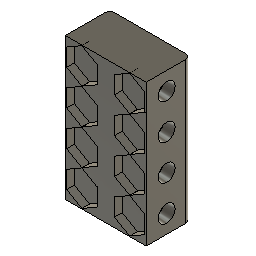
frame_rail_connector_block (Autodesk Fusion 360 archive; units mm, degrees)
design "frame connector block" references "2u(ish) rail"
Autodesk Fusion 360 part; units mm, degrees
imported_body "Derived Base Feature1" makes body 1
other "ExternalDerived1"
sketch "Sketch1" plane through (0, 0, 0) normal (0, 0, 1) x (1, 0, 0)
  arc A0 (4.25, 3.5) -> (5.75, 2) centre (5.75, 3.5) ccw
  line L0 (4.25, 3.5) -> (4.25, 14.875)
  line L1 (26, 2) -> (5.75, 2)
  arc A1 (26, 2) -> (27.5, 3.5) centre (26, 3.5) ccw
  line L2 (27.75, 3.5) -> (27.75, 14.875)
  line L3 (27.5, 14.875) -> (27.5, 3.5)
  line L4 (5.75, 14.875) -> (26, 14.875)
  line L5 (27.5, 13.375) -> (27.5, 3.5)
  line L6 (26, 2) -> (5.75, 2)
  line L7 (4.25, 3.5) -> (4.25, 13.375)
  arc A2 (4.25, 3.5) -> (5.75, 2) centre (5.75, 3.5) ccw
  arc A3 (26, 2) -> (27.5, 3.5) centre (26, 3.5) ccw
  arc A4 (5.75, 14.875) -> (4.25, 13.375) centre (5.75, 13.375) ccw
  arc A5 (27.5, 13.375) -> (26, 14.875) centre (26, 13.375) ccw
  arc A6 (27.4, 13.375) -> (26, 14.775) centre (26, 13.375) ccw
  line L8 (5.75, 14.775) -> (26, 14.775)
  arc A7 (5.75, 14.775) -> (4.35, 13.375) centre (5.75, 13.375) ccw
  line L9 (4.35, 3.5) -> (4.35, 13.375)
  arc A8 (4.35, 3.5) -> (5.75, 2.1) centre (5.75, 3.5) ccw
  line L10 (26, 2.1) -> (5.75, 2.1)
  arc A9 (26, 2.1) -> (27.4, 3.5) centre (26, 3.5) ccw
  line L11 (27.4, 13.375) -> (27.4, 3.5)
  dimension "d12" = 1.5
  dimension "d13" = 1.5
  dimension "d14" = 1.5
  dimension "d15" = 1.5
  dimension "d16" = 0.1
  constraint horizontal L4
  constraint vertical L5
  constraint horizontal L6
  constraint vertical L7
  constraint tangent L6 A2
  constraint tangent L7 A2
  constraint tangent L5 A3
  constraint tangent L6 A3
  constraint tangent L4 A4
  constraint tangent L7 A4
  constraint tangent L4 A5
  constraint tangent L5 A5
  measures "d12" radius of A2
  measures "d13" radius of A3
  measures "d14" radius of A4
  measures "d15" radius of A5
extrude "Extrude1" add sketch "Sketch1" along normal blind 40.25 separate body contours A6 L8 A7 L9 A8 L10 A9 L11 makes body 2
sketch "Sketch2" plane through (4.25, 0, 0) normal (1, 0, 0) x (0, 1, 0)
  line L0 (3.5, 0.25) -> (14.875, 0.25)
  line L1 (14.875, 0.25) -> (14.875, 130.5625)
  line L2 (14.875, 130.5625) -> (3.5, 130.5625)
  line L3 (3.5, 130.5625) -> (3.5, 0.25)
  line L4 (5.6281, 35.2188) -> (6.7828, 37.2188)
  line L5 (6.7828, 37.2188) -> (9.0922, 37.2188)
  line L6 (9.0922, 37.2188) -> (10.2469, 35.2188)
  line L7 (10.2469, 35.2188) -> (9.0922, 33.2188)
  line L8 (9.0922, 33.2188) -> (6.7828, 33.2188)
  line L9 (6.7828, 33.2188) -> (5.6281, 35.2188)
  line L10 (5.6281, 75.4688) -> (6.7828, 77.4688)
  line L11 (6.7828, 77.4688) -> (9.0922, 77.4688)
  line L12 (9.0922, 77.4688) -> (10.2469, 75.4688)
  line L13 (10.2469, 75.4688) -> (9.0922, 73.4688)
  line L14 (9.0922, 73.4688) -> (6.7828, 73.4688)
  line L15 (6.7828, 73.4688) -> (5.6281, 75.4688)
  line L16 (5.6281, 115.7188) -> (6.7828, 117.7188)
  line L17 (6.7828, 117.7188) -> (9.0922, 117.7188)
  line L18 (9.0922, 117.7188) -> (10.2469, 115.7188)
  line L19 (10.2469, 115.7188) -> (9.0922, 113.7188)
  line L20 (9.0922, 113.7188) -> (6.7828, 113.7188)
  line L21 (6.7828, 113.7188) -> (5.6281, 115.7188)
  line L22 (5.6281, 125.7813) -> (6.7828, 127.7813)
  line L23 (6.7828, 127.7813) -> (9.0922, 127.7813)
  line L24 (9.0922, 127.7813) -> (10.2469, 125.7813)
  line L25 (10.2469, 125.7813) -> (9.0922, 123.7813)
  line L26 (9.0922, 123.7813) -> (6.7828, 123.7813)
  line L27 (6.7828, 123.7813) -> (5.6281, 125.7813)
  line L28 (5.6281, 85.5313) -> (6.7828, 87.5313)
  line L29 (6.7828, 87.5313) -> (9.0922, 87.5313)
  line L30 (9.0922, 87.5313) -> (10.2469, 85.5313)
  line L31 (10.2469, 85.5313) -> (9.0922, 83.5313)
  line L32 (9.0922, 83.5313) -> (6.7828, 83.5313)
  line L33 (6.7828, 83.5313) -> (5.6281, 85.5313)
  line L34 (5.6281, 45.2813) -> (6.7828, 47.2813)
  line L35 (6.7828, 47.2813) -> (9.0922, 47.2813)
  line L36 (9.0922, 47.2813) -> (10.2469, 45.2813)
  line L37 (10.2469, 45.2813) -> (9.0922, 43.2813)
  line L38 (9.0922, 43.2813) -> (6.7828, 43.2813)
  line L39 (6.7828, 43.2813) -> (5.6281, 45.2813)
  line L40 (5.6281, 25.1563) -> (6.7828, 27.1563)
  line L41 (6.7828, 27.1563) -> (9.0922, 27.1563)
  line L42 (9.0922, 27.1563) -> (10.2469, 25.1563)
  line L43 (10.2469, 25.1563) -> (9.0922, 23.1563)
  line L44 (9.0922, 23.1563) -> (6.7828, 23.1563)
  line L45 (6.7828, 23.1563) -> (5.6281, 25.1563)
  line L46 (5.6281, 65.4063) -> (6.7828, 67.4063)
  line L47 (6.7828, 67.4063) -> (9.0922, 67.4063)
  line L48 (9.0922, 67.4063) -> (10.2469, 65.4063)
  line L49 (10.2469, 65.4063) -> (9.0922, 63.4063)
  line L50 (9.0922, 63.4063) -> (6.7828, 63.4063)
  line L51 (6.7828, 63.4063) -> (5.6281, 65.4063)
  line L52 (5.6281, 105.6563) -> (6.7828, 107.6563)
  line L53 (6.7828, 107.6563) -> (9.0922, 107.6563)
  line L54 (9.0922, 107.6563) -> (10.2469, 105.6563)
  line L55 (10.2469, 105.6563) -> (9.0922, 103.6563)
  line L56 (9.0922, 103.6563) -> (6.7828, 103.6563)
  line L57 (6.7828, 103.6563) -> (5.6281, 105.6563)
  line L58 (10.2469, 5.0313) -> (9.0922, 3.0313)
  line L59 (9.0922, 3.0313) -> (6.7828, 3.0313)
  line L60 (6.7828, 3.0313) -> (5.6281, 5.0313)
  line L61 (5.6281, 5.0313) -> (6.7828, 7.0313)
  line L62 (6.7828, 7.0313) -> (9.0922, 7.0313)
  line L63 (9.0922, 7.0313) -> (10.2469, 5.0313)
  line L64 (5.6281, 95.5938) -> (6.7828, 97.5938)
  line L65 (6.7828, 97.5938) -> (9.0922, 97.5938)
  line L66 (9.0922, 97.5938) -> (10.2469, 95.5938)
  line L67 (10.2469, 95.5938) -> (9.0922, 93.5938)
  line L68 (9.0922, 93.5938) -> (6.7828, 93.5938)
  line L69 (6.7828, 93.5938) -> (5.6281, 95.5938)
  line L70 (5.6281, 55.3438) -> (6.7828, 57.3438)
  line L71 (6.7828, 57.3438) -> (9.0922, 57.3438)
  line L72 (9.0922, 57.3438) -> (10.2469, 55.3438)
  line L73 (10.2469, 55.3438) -> (9.0922, 53.3438)
  line L74 (9.0922, 53.3438) -> (6.7828, 53.3438)
  line L75 (6.7828, 53.3438) -> (5.6281, 55.3438)
  line L76 (5.6281, 15.0938) -> (6.7828, 17.0938)
  line L77 (6.7828, 17.0938) -> (9.0922, 17.0938)
  line L78 (9.0922, 17.0938) -> (10.2469, 15.0938)
  line L79 (10.2469, 15.0938) -> (9.0922, 13.0938)
  line L80 (9.0922, 13.0938) -> (6.7828, 13.0938)
  line L81 (6.7828, 13.0938) -> (5.6281, 15.0938)
  line L82 (6.7828, 17.0938) -> (5.6281, 15.0938)
  line L83 (5.6281, 15.0938) -> (6.7828, 13.0938)
  line L84 (6.7828, 13.0938) -> (9.0922, 13.0938)
  line L85 (9.0922, 13.0938) -> (10.2469, 15.0938)
  line L86 (10.2469, 15.0938) -> (9.0922, 17.0938)
  line L87 (9.0922, 17.0938) -> (6.7828, 17.0938)
  line L88 (6.7828, 57.3438) -> (5.6281, 55.3438)
  line L89 (5.6281, 55.3438) -> (6.7828, 53.3438)
  line L90 (6.7828, 53.3438) -> (9.0922, 53.3438)
  line L91 (9.0922, 53.3438) -> (10.2469, 55.3438)
  line L92 (10.2469, 55.3438) -> (9.0922, 57.3438)
  line L93 (9.0922, 57.3438) -> (6.7828, 57.3438)
  line L94 (6.7828, 97.5938) -> (5.6281, 95.5938)
  line L95 (5.6281, 95.5938) -> (6.7828, 93.5938)
  line L96 (6.7828, 93.5938) -> (9.0922, 93.5938)
  line L97 (9.0922, 93.5938) -> (10.2469, 95.5938)
  line L98 (10.2469, 95.5938) -> (9.0922, 97.5938)
  line L99 (9.0922, 97.5938) -> (6.7828, 97.5938)
  line L100 (9.0922, 3.0313) -> (10.2469, 5.0313)
  line L101 (10.2469, 5.0313) -> (9.0922, 7.0313)
  line L102 (9.0922, 7.0313) -> (6.7828, 7.0313)
  line L103 (6.7828, 7.0313) -> (5.6281, 5.0313)
  line L104 (5.6281, 5.0313) -> (6.7828, 3.0313)
  line L105 (6.7828, 3.0313) -> (9.0922, 3.0313)
  line L106 (6.7828, 107.6563) -> (5.6281, 105.6563)
  line L107 (5.6281, 105.6563) -> (6.7828, 103.6563)
  line L108 (6.7828, 103.6563) -> (9.0922, 103.6563)
  line L109 (9.0922, 103.6563) -> (10.2469, 105.6563)
  line L110 (10.2469, 105.6563) -> (9.0922, 107.6563)
  line L111 (9.0922, 107.6563) -> (6.7828, 107.6563)
  line L112 (6.7828, 67.4063) -> (5.6281, 65.4063)
  line L113 (5.6281, 65.4063) -> (6.7828, 63.4063)
  line L114 (6.7828, 63.4063) -> (9.0922, 63.4063)
  line L115 (9.0922, 63.4063) -> (10.2469, 65.4063)
  line L116 (10.2469, 65.4063) -> (9.0922, 67.4063)
  line L117 (9.0922, 67.4063) -> (6.7828, 67.4063)
  line L118 (6.7828, 27.1563) -> (5.6281, 25.1563)
  line L119 (5.6281, 25.1563) -> (6.7828, 23.1563)
  line L120 (6.7828, 23.1563) -> (9.0922, 23.1563)
  line L121 (9.0922, 23.1563) -> (10.2469, 25.1563)
  line L122 (10.2469, 25.1563) -> (9.0922, 27.1563)
  line L123 (9.0922, 27.1563) -> (6.7828, 27.1563)
  line L124 (6.7828, 47.2813) -> (5.6281, 45.2813)
  line L125 (5.6281, 45.2813) -> (6.7828, 43.2813)
  line L126 (6.7828, 43.2813) -> (9.0922, 43.2813)
  line L127 (9.0922, 43.2813) -> (10.2469, 45.2813)
  line L128 (10.2469, 45.2813) -> (9.0922, 47.2813)
  line L129 (9.0922, 47.2813) -> (6.7828, 47.2813)
  line L130 (6.7828, 87.5313) -> (5.6281, 85.5313)
  line L131 (5.6281, 85.5313) -> (6.7828, 83.5313)
  line L132 (6.7828, 83.5313) -> (9.0922, 83.5313)
  line L133 (9.0922, 83.5313) -> (10.2469, 85.5313)
  line L134 (10.2469, 85.5313) -> (9.0922, 87.5313)
  line L135 (9.0922, 87.5313) -> (6.7828, 87.5313)
  line L136 (6.7828, 127.7813) -> (5.6281, 125.7813)
  line L137 (5.6281, 125.7813) -> (6.7828, 123.7813)
  line L138 (6.7828, 123.7813) -> (9.0922, 123.7813)
  line L139 (9.0922, 123.7813) -> (10.2469, 125.7813)
  line L140 (10.2469, 125.7813) -> (9.0922, 127.7813)
  line L141 (9.0922, 127.7813) -> (6.7828, 127.7813)
  line L142 (6.7828, 117.7188) -> (5.6281, 115.7188)
  line L143 (5.6281, 115.7188) -> (6.7828, 113.7188)
  line L144 (6.7828, 113.7188) -> (9.0922, 113.7188)
  line L145 (9.0922, 113.7188) -> (10.2469, 115.7188)
  line L146 (10.2469, 115.7188) -> (9.0922, 117.7188)
  line L147 (9.0922, 117.7188) -> (6.7828, 117.7188)
  line L148 (6.7828, 77.4688) -> (5.6281, 75.4688)
  line L149 (5.6281, 75.4688) -> (6.7828, 73.4688)
  line L150 (6.7828, 73.4688) -> (9.0922, 73.4688)
  line L151 (9.0922, 73.4688) -> (10.2469, 75.4688)
  line L152 (10.2469, 75.4688) -> (9.0922, 77.4688)
  line L153 (9.0922, 77.4688) -> (6.7828, 77.4688)
  line L154 (6.7828, 37.2188) -> (5.6281, 35.2188)
  line L155 (5.6281, 35.2188) -> (6.7828, 33.2188)
  line L156 (6.7828, 33.2188) -> (9.0922, 33.2188)
  line L157 (9.0922, 33.2188) -> (10.2469, 35.2188)
  line L158 (10.2469, 35.2188) -> (9.0922, 37.2188)
  line L159 (9.0922, 37.2188) -> (6.7828, 37.2188)
  line L160 (14.875, 0.25) -> (1, 0.25)
  line L161 (1, 0.25) -> (1, 130.5625)
  line L162 (1, 130.5625) -> (14.875, 130.5625)
  line L163 (14.875, 130.5625) -> (14.875, 0.25)
  circle A0 centre (7.9375, 5.0313) radius 2
  circle A1 centre (7.9375, 15.0938) radius 2
  circle A2 centre (7.9375, 25.1563) radius 2
  circle A3 centre (7.9375, 35.2188) radius 2
  dimension "d19" = 4
  dimension "d20" = 4
  dimension "d21" = 4
  dimension "d22" = 4
  measures "d19" diameter of A0
  measures "d20" diameter of A1
  measures "d21" diameter of A2
  measures "d22" diameter of A3
sketch "Sketch3" plane through (27.4, 0, 0) normal (1, 0, 0) x (0, 1, 0)
  line L0 (3.5, 0) -> (13.375, 0)
  line L1 (13.375, 0) -> (13.375, 40.25)
  line L2 (13.375, 40.25) -> (3.5, 40.25)
  line L3 (3.5, 40.25) -> (3.5, 0)
  line L4 (5.6281, 35.2188) -> (6.7828, 37.2188)
  line L5 (6.7828, 37.2188) -> (9.0922, 37.2188)
  line L6 (9.0922, 37.2188) -> (10.2469, 35.2188)
  line L7 (10.2469, 35.2188) -> (9.0922, 33.2188)
  line L8 (9.0922, 33.2188) -> (6.7828, 33.2188)
  line L9 (6.7828, 33.2188) -> (5.6281, 35.2188)
  line L10 (5.6281, 75.4688) -> (6.7828, 77.4688)
  line L11 (6.7828, 77.4688) -> (9.0922, 77.4688)
  line L12 (9.0922, 77.4688) -> (10.2469, 75.4688)
  line L13 (10.2469, 75.4688) -> (9.0922, 73.4688)
  line L14 (9.0922, 73.4688) -> (6.7828, 73.4688)
  line L15 (6.7828, 73.4688) -> (5.6281, 75.4688)
  line L16 (5.6281, 115.7188) -> (6.7828, 117.7188)
  line L17 (6.7828, 117.7188) -> (9.0922, 117.7188)
  line L18 (9.0922, 117.7188) -> (10.2469, 115.7188)
  line L19 (10.2469, 115.7188) -> (9.0922, 113.7188)
  line L20 (9.0922, 113.7188) -> (6.7828, 113.7188)
  line L21 (6.7828, 113.7188) -> (5.6281, 115.7188)
  line L22 (5.6281, 125.7813) -> (6.7828, 127.7813)
  line L23 (6.7828, 127.7813) -> (9.0922, 127.7813)
  line L24 (9.0922, 127.7813) -> (10.2469, 125.7813)
  line L25 (10.2469, 125.7813) -> (9.0922, 123.7813)
  line L26 (9.0922, 123.7813) -> (6.7828, 123.7813)
  line L27 (6.7828, 123.7813) -> (5.6281, 125.7813)
  line L28 (5.6281, 85.5313) -> (6.7828, 87.5313)
  line L29 (6.7828, 87.5313) -> (9.0922, 87.5313)
  line L30 (9.0922, 87.5313) -> (10.2469, 85.5313)
  line L31 (10.2469, 85.5313) -> (9.0922, 83.5313)
  line L32 (9.0922, 83.5313) -> (6.7828, 83.5313)
  line L33 (6.7828, 83.5313) -> (5.6281, 85.5313)
  line L34 (5.6281, 45.2813) -> (6.7828, 47.2813)
  line L35 (6.7828, 47.2813) -> (9.0922, 47.2813)
  line L36 (9.0922, 47.2813) -> (10.2469, 45.2813)
  line L37 (10.2469, 45.2813) -> (9.0922, 43.2813)
  line L38 (9.0922, 43.2813) -> (6.7828, 43.2813)
  line L39 (6.7828, 43.2813) -> (5.6281, 45.2813)
  line L40 (5.6281, 25.1563) -> (6.7828, 27.1563)
  line L41 (6.7828, 27.1563) -> (9.0922, 27.1563)
  line L42 (9.0922, 27.1563) -> (10.2469, 25.1563)
  line L43 (10.2469, 25.1563) -> (9.0922, 23.1563)
  line L44 (9.0922, 23.1563) -> (6.7828, 23.1563)
  line L45 (6.7828, 23.1563) -> (5.6281, 25.1563)
  line L46 (5.6281, 65.4063) -> (6.7828, 67.4063)
  line L47 (6.7828, 67.4063) -> (9.0922, 67.4063)
  line L48 (9.0922, 67.4063) -> (10.2469, 65.4063)
  line L49 (10.2469, 65.4063) -> (9.0922, 63.4063)
  line L50 (9.0922, 63.4063) -> (6.7828, 63.4063)
  line L51 (6.7828, 63.4063) -> (5.6281, 65.4063)
  line L52 (5.6281, 105.6563) -> (6.7828, 107.6563)
  line L53 (6.7828, 107.6563) -> (9.0922, 107.6563)
  line L54 (9.0922, 107.6563) -> (10.2469, 105.6563)
  line L55 (10.2469, 105.6563) -> (9.0922, 103.6563)
  line L56 (9.0922, 103.6563) -> (6.7828, 103.6563)
  line L57 (6.7828, 103.6563) -> (5.6281, 105.6563)
  line L58 (10.2469, 5.0313) -> (9.0922, 3.0313)
  line L59 (9.0922, 3.0313) -> (6.7828, 3.0313)
  line L60 (6.7828, 3.0313) -> (5.6281, 5.0313)
  line L61 (5.6281, 5.0313) -> (6.7828, 7.0313)
  line L62 (6.7828, 7.0313) -> (9.0922, 7.0313)
  line L63 (9.0922, 7.0313) -> (10.2469, 5.0313)
  line L64 (5.6281, 95.5938) -> (6.7828, 97.5938)
  line L65 (6.7828, 97.5938) -> (9.0922, 97.5938)
  line L66 (9.0922, 97.5938) -> (10.2469, 95.5938)
  line L67 (10.2469, 95.5938) -> (9.0922, 93.5938)
  line L68 (9.0922, 93.5938) -> (6.7828, 93.5938)
  line L69 (6.7828, 93.5938) -> (5.6281, 95.5938)
  line L70 (5.6281, 55.3438) -> (6.7828, 57.3438)
  line L71 (6.7828, 57.3438) -> (9.0922, 57.3438)
  line L72 (9.0922, 57.3438) -> (10.2469, 55.3438)
  line L73 (10.2469, 55.3438) -> (9.0922, 53.3438)
  line L74 (9.0922, 53.3438) -> (6.7828, 53.3438)
  line L75 (6.7828, 53.3438) -> (5.6281, 55.3438)
  line L76 (5.6281, 15.0938) -> (6.7828, 17.0938)
  line L77 (6.7828, 17.0938) -> (9.0922, 17.0938)
  line L78 (9.0922, 17.0938) -> (10.2469, 15.0938)
  line L79 (10.2469, 15.0938) -> (9.0922, 13.0938)
  line L80 (9.0922, 13.0938) -> (6.7828, 13.0938)
  line L81 (6.7828, 13.0938) -> (5.6281, 15.0938)
  line L82 (1, 0.25) -> (14.875, 0.25)
  line L83 (14.875, 0.25) -> (14.875, 130.5625)
  line L84 (14.875, 130.5625) -> (1, 130.5625)
  line L85 (1, 130.5625) -> (1, 0.25)
  circle A0 centre (7.9375, 5.0313) radius 2
  circle A1 centre (7.9375, 15.0938) radius 2
  circle A2 centre (7.9375, 35.2188) radius 2
  circle A3 centre (7.9375, 25.1563) radius 2
  dimension "d23" = 4
  dimension "d24" = 4
  dimension "d25" = 4
  dimension "d26" = 4
  measures "d23" diameter of A0
  measures "d24" diameter of A1
  measures "d25" diameter of A2
  measures "d26" diameter of A3
hole "Hole1" at (27.4, 7.9375, 5.0313) at (27.4, 7.9375, 15.0938) at (27.4, 7.9375, 25.1563) at (27.4, 7.9375, 35.2188) direction (-1, 0, 0) diameter 4.1 depth 8 tip angle 180 counterbore diameter 4.8 counterbore depth 3 bodies 2
sketch "Sketch4" plane through (4.35, 0, 0) normal (-1, 0, 0) x (0, -1, 0)
  line L0 (-13.375, 0) -> (-3.5, 0)
  line L1 (-3.5, 0) -> (-3.5, 40.25)
  line L2 (-3.5, 40.25) -> (-13.375, 40.25)
  line L3 (-13.375, 40.25) -> (-13.375, 0)
  line L4 (-6.7828, 17.0938) -> (-5.6281, 15.0938)
  line L5 (-5.6281, 15.0938) -> (-6.7828, 13.0938)
  line L6 (-6.7828, 13.0938) -> (-9.0922, 13.0938)
  line L7 (-9.0922, 13.0938) -> (-10.2469, 15.0938)
  line L8 (-10.2469, 15.0938) -> (-9.0922, 17.0938)
  line L9 (-9.0922, 17.0938) -> (-6.7828, 17.0938)
  line L10 (-6.7828, 57.3438) -> (-5.6281, 55.3438)
  line L11 (-5.6281, 55.3438) -> (-6.7828, 53.3438)
  line L12 (-6.7828, 53.3438) -> (-9.0922, 53.3438)
  line L13 (-9.0922, 53.3438) -> (-10.2469, 55.3438)
  line L14 (-10.2469, 55.3438) -> (-9.0922, 57.3438)
  line L15 (-9.0922, 57.3438) -> (-6.7828, 57.3438)
  line L16 (-6.7828, 97.5938) -> (-5.6281, 95.5938)
  line L17 (-5.6281, 95.5938) -> (-6.7828, 93.5938)
  line L18 (-6.7828, 93.5938) -> (-9.0922, 93.5938)
  line L19 (-9.0922, 93.5938) -> (-10.2469, 95.5938)
  line L20 (-10.2469, 95.5938) -> (-9.0922, 97.5938)
  line L21 (-9.0922, 97.5938) -> (-6.7828, 97.5938)
  line L22 (-9.0922, 3.0313) -> (-10.2469, 5.0313)
  line L23 (-10.2469, 5.0313) -> (-9.0922, 7.0313)
  line L24 (-9.0922, 7.0313) -> (-6.7828, 7.0313)
  line L25 (-6.7828, 7.0313) -> (-5.6281, 5.0313)
  line L26 (-5.6281, 5.0313) -> (-6.7828, 3.0313)
  line L27 (-6.7828, 3.0313) -> (-9.0922, 3.0313)
  line L28 (-6.7828, 107.6563) -> (-5.6281, 105.6563)
  line L29 (-5.6281, 105.6563) -> (-6.7828, 103.6563)
  line L30 (-6.7828, 103.6563) -> (-9.0922, 103.6563)
  line L31 (-9.0922, 103.6563) -> (-10.2469, 105.6563)
  line L32 (-10.2469, 105.6563) -> (-9.0922, 107.6563)
  line L33 (-9.0922, 107.6563) -> (-6.7828, 107.6563)
  line L34 (-6.7828, 67.4063) -> (-5.6281, 65.4063)
  line L35 (-5.6281, 65.4063) -> (-6.7828, 63.4063)
  line L36 (-6.7828, 63.4063) -> (-9.0922, 63.4063)
  line L37 (-9.0922, 63.4063) -> (-10.2469, 65.4063)
  line L38 (-10.2469, 65.4063) -> (-9.0922, 67.4063)
  line L39 (-9.0922, 67.4063) -> (-6.7828, 67.4063)
  line L40 (-6.7828, 27.1563) -> (-5.6281, 25.1563)
  line L41 (-5.6281, 25.1563) -> (-6.7828, 23.1563)
  line L42 (-6.7828, 23.1563) -> (-9.0922, 23.1563)
  line L43 (-9.0922, 23.1563) -> (-10.2469, 25.1563)
  line L44 (-10.2469, 25.1563) -> (-9.0922, 27.1563)
  line L45 (-9.0922, 27.1563) -> (-6.7828, 27.1563)
  line L46 (-6.7828, 47.2813) -> (-5.6281, 45.2813)
  line L47 (-5.6281, 45.2813) -> (-6.7828, 43.2813)
  line L48 (-6.7828, 43.2813) -> (-9.0922, 43.2813)
  line L49 (-9.0922, 43.2813) -> (-10.2469, 45.2813)
  line L50 (-10.2469, 45.2813) -> (-9.0922, 47.2813)
  line L51 (-9.0922, 47.2813) -> (-6.7828, 47.2813)
  line L52 (-6.7828, 87.5313) -> (-5.6281, 85.5313)
  line L53 (-5.6281, 85.5313) -> (-6.7828, 83.5313)
  line L54 (-6.7828, 83.5313) -> (-9.0922, 83.5313)
  line L55 (-9.0922, 83.5313) -> (-10.2469, 85.5313)
  line L56 (-10.2469, 85.5313) -> (-9.0922, 87.5313)
  line L57 (-9.0922, 87.5313) -> (-6.7828, 87.5313)
  line L58 (-6.7828, 127.7813) -> (-5.6281, 125.7813)
  line L59 (-5.6281, 125.7813) -> (-6.7828, 123.7813)
  line L60 (-6.7828, 123.7813) -> (-9.0922, 123.7813)
  line L61 (-9.0922, 123.7813) -> (-10.2469, 125.7813)
  line L62 (-10.2469, 125.7813) -> (-9.0922, 127.7813)
  line L63 (-9.0922, 127.7813) -> (-6.7828, 127.7813)
  line L64 (-6.7828, 117.7188) -> (-5.6281, 115.7188)
  line L65 (-5.6281, 115.7188) -> (-6.7828, 113.7188)
  line L66 (-6.7828, 113.7188) -> (-9.0922, 113.7188)
  line L67 (-9.0922, 113.7188) -> (-10.2469, 115.7188)
  line L68 (-10.2469, 115.7188) -> (-9.0922, 117.7188)
  line L69 (-9.0922, 117.7188) -> (-6.7828, 117.7188)
  line L70 (-6.7828, 77.4688) -> (-5.6281, 75.4688)
  line L71 (-5.6281, 75.4688) -> (-6.7828, 73.4688)
  line L72 (-6.7828, 73.4688) -> (-9.0922, 73.4688)
  line L73 (-9.0922, 73.4688) -> (-10.2469, 75.4688)
  line L74 (-10.2469, 75.4688) -> (-9.0922, 77.4688)
  line L75 (-9.0922, 77.4688) -> (-6.7828, 77.4688)
  line L76 (-6.7828, 37.2188) -> (-5.6281, 35.2188)
  line L77 (-5.6281, 35.2188) -> (-6.7828, 33.2188)
  line L78 (-6.7828, 33.2188) -> (-9.0922, 33.2188)
  line L79 (-9.0922, 33.2188) -> (-10.2469, 35.2188)
  line L80 (-10.2469, 35.2188) -> (-9.0922, 37.2188)
  line L81 (-9.0922, 37.2188) -> (-6.7828, 37.2188)
  line L82 (-14.875, 0.25) -> (-1, 0.25)
  line L83 (-1, 0.25) -> (-1, 130.5625)
  line L84 (-1, 130.5625) -> (-14.875, 130.5625)
  line L85 (-14.875, 130.5625) -> (-14.875, 0.25)
  circle A0 centre (-7.9375, 5.0313) radius 2
  circle A1 centre (-7.9375, 15.0938) radius 2
  circle A2 centre (-7.9375, 25.1563) radius 2
  circle A3 centre (-7.9375, 35.2188) radius 2
  dimension "d32" = 4
  dimension "d33" = 4
  dimension "d34" = 4
  dimension "d35" = 4
  measures "d32" diameter of A0
  measures "d33" diameter of A1
  measures "d34" diameter of A2
  measures "d35" diameter of A3
hole "Hole2" at (4.35, 7.9375, 35.2188) at (4.35, 7.9375, 25.1563) at (4.35, 7.9375, 15.0938) at (4.35, 7.9375, 5.0313) direction (1, 0, 0) diameter 4.1 depth 8 tip angle 180 counterbore diameter 4.8 counterbore depth 3 bodies 2
chamfer "Chamfer1" distance 3 distance2 0.3 4 edges at (7.35, 10.1751, 36.0867) (7.35, 10.1751, 26.0242) (7.35, 10.1751, 15.9617) (7.35, 10.1751, 5.8992) measured on face at (5.35, 8.0571, 37.6158) measured on face at (5.35, 8.0571, 27.5533) measured on face at (5.35, 8.0571, 17.4908) measured on face at (5.35, 8.0571, 7.4283) on bodies 2
chamfer "Chamfer1" distance 3 distance2 0.3 4 edges at (24.4, 5.6999, 36.0867) (24.4, 5.6999, 26.0242) (24.4, 5.6999, 15.9617) (24.4, 5.6999, 5.8992) measured on face at (26.4, 8.0571, 32.8218) measured on face at (26.4, 8.0571, 22.7593) measured on face at (26.4, 8.0571, 12.6968) measured on face at (26.4, 8.0571, 2.6343) on bodies 2
fillet "Fillet1" [suppressed]
sketch "Sketch5" plane through (0, 2.1, 0) normal (0, -1, 0) x (1, 0, 0)
  line L0 (26, 0) -> (26, 40.25)
  line L1 (5.75, 40.25) -> (5.75, 0)
  line L2 (1, 0.25) -> (30.75, 0.25)
  line L3 (30.75, 0.25) -> (30.75, 130.5625)
  line L4 (30.75, 130.5625) -> (1, 130.5625)
  line L5 (1, 130.5625) -> (1, 0.25)
  circle A0 centre (9.0625, 5.0313) radius 3.1
  circle A1 centre (9.0625, 55.3438) radius 3.1
  circle A2 centre (22.6875, 15.0938) radius 3.1
  circle A3 centre (9.0625, 125.7813) radius 3.1
  circle A4 centre (22.6875, 105.6563) radius 3.1
  circle A5 centre (22.6875, 5.0313) radius 3.1
  circle A6 centre (22.6875, 65.4063) radius 3.1
  circle A7 centre (9.0625, 45.2813) radius 3.1
  circle A8 centre (22.6875, 125.7813) radius 3.1
  circle A9 centre (9.0625, 75.4688) radius 3.1
  circle A10 centre (9.0625, 25.1563) radius 3.1
  circle A11 centre (9.0625, 15.0938) radius 3.1
  circle A12 centre (22.6875, 35.2188) radius 3.1
  circle A13 centre (22.6875, 95.5938) radius 3.1
  circle A14 centre (22.6875, 55.3438) radius 3.1
  circle A15 centre (22.6875, 85.5313) radius 3.1
  circle A16 centre (9.0625, 95.5938) radius 3.1
  circle A17 centre (9.0625, 35.2188) radius 3.1
  circle A18 centre (22.6875, 115.7188) radius 3.1
  circle A19 centre (22.6875, 75.4688) radius 3.1
  circle A20 centre (9.0625, 105.6563) radius 3.1
  circle A21 centre (9.0625, 115.7188) radius 3.1
  circle A22 centre (9.0625, 85.5313) radius 3.1
  circle A23 centre (22.6875, 25.1563) radius 3.1
  circle A24 centre (9.0625, 65.4063) radius 3.1
  circle A25 centre (22.6875, 45.2813) radius 3.1
  line L6 (9.0625, 30.2188) -> (13.3926, 32.7188)
  line L7 (13.3926, 32.7188) -> (13.3926, 37.7188)
  line L8 (13.3926, 37.7188) -> (9.0625, 40.2188)
  line L9 (9.0625, 40.2188) -> (4.7324, 37.7188)
  line L10 (4.7324, 37.7188) -> (4.7324, 32.7188)
  line L11 (4.7324, 32.7188) -> (9.0625, 30.2188)
  line L12 (22.6875, 30.2188) -> (27.0176, 32.7188)
  line L13 (27.0176, 32.7188) -> (27.0176, 37.7188)
  line L14 (27.0176, 37.7188) -> (22.6875, 40.2188)
  line L15 (22.6875, 40.2188) -> (18.3574, 37.7188)
  line L16 (18.3574, 37.7188) -> (18.3574, 32.7188)
  line L17 (18.3574, 32.7188) -> (22.6875, 30.2188)
  line L18 (22.6905, 30.1563) -> (18.3589, 27.6589)
  line L19 (18.3589, 27.6589) -> (18.3559, 22.6589)
  line L20 (18.3559, 22.6589) -> (22.6845, 20.1563)
  line L21 (22.6845, 20.1563) -> (27.0161, 22.6537)
  line L22 (27.0161, 22.6537) -> (27.0191, 27.6537)
  line L23 (27.0191, 27.6537) -> (22.6905, 30.1563)
  line L24 (9.0625, 30.1563) -> (4.7324, 27.6563)
  line L25 (4.7324, 27.6563) -> (4.7324, 22.6563)
  line L26 (4.7324, 22.6563) -> (9.0625, 20.1563)
  line L27 (9.0625, 20.1563) -> (13.3926, 22.6563)
  line L28 (13.3926, 22.6563) -> (13.3926, 27.6563)
  line L29 (13.3926, 27.6563) -> (9.0625, 30.1563)
  line L30 (9.0625, 10.0938) -> (13.3926, 12.5938)
  line L31 (13.3926, 12.5938) -> (13.3926, 17.5938)
  line L32 (13.3926, 17.5938) -> (9.0625, 20.0938)
  line L33 (9.0625, 20.0938) -> (4.7324, 17.5938)
  line L34 (4.7324, 17.5938) -> (4.7324, 12.5938)
  line L35 (4.7324, 12.5938) -> (9.0625, 10.0938)
  line L36 (22.6875, 10.0938) -> (27.0176, 12.5938)
  line L37 (27.0176, 12.5938) -> (27.0176, 17.5938)
  line L38 (27.0176, 17.5938) -> (22.6875, 20.0938)
  line L39 (22.6875, 20.0938) -> (18.3574, 17.5938)
  line L40 (18.3574, 17.5938) -> (18.3574, 12.5938)
  line L41 (18.3574, 12.5938) -> (22.6875, 10.0938)
  line L42 (22.6875, 0.0313) -> (27.0176, 2.5313)
  line L43 (27.0176, 2.5313) -> (27.0176, 7.5313)
  line L44 (27.0176, 7.5313) -> (22.6875, 10.0313)
  line L45 (22.6875, 10.0313) -> (18.3574, 7.5313)
  line L46 (18.3574, 7.5313) -> (18.3574, 2.5313)
  line L47 (18.3574, 2.5313) -> (22.6875, 0.0313)
  line L48 (9.0625, 0.0313) -> (13.3926, 2.5313)
  line L49 (13.3926, 2.5313) -> (13.3926, 7.5313)
  line L50 (13.3926, 7.5313) -> (9.0625, 10.0313)
  line L51 (9.0625, 10.0313) -> (4.7324, 7.5313)
  line L52 (4.7324, 7.5313) -> (4.7324, 2.5313)
  line L53 (4.7324, 2.5313) -> (9.0625, 0.0313)
  line L54 (5.75, 0) -> (26, 0)
  line L55 (26, 40.25) -> (5.75, 40.25)
  point P0 (9.0625, 35.2188)
  point P1 (22.6875, 35.2188)
  point P2 (22.6875, 25.1563)
  point P3 (9.0625, 25.1563)
  point P4 (9.0625, 15.0938)
  point P5 (22.6875, 15.0938)
  point P6 (22.6875, 5.0313)
  point P7 (9.0625, 5.0313)
  dimension "d49" = 5
  dimension "d50" = 5
  dimension "d51" = 5
  dimension "d52" = 5
  dimension "d53" = 5
  dimension "d54" = 5
  dimension "d55" = 5
  dimension "d56" = 5
  constraint coincident P0 A17.centre
  constraint coincident P1 A12.centre
  constraint coincident P2 A23.centre
  constraint coincident P3 A10.centre
  constraint coincident P4 A11.centre
  constraint coincident P5 A2.centre
  constraint coincident P6 A5.centre
  constraint coincident P7 A0.centre
  measures "d49" distance of L6.start P0
  measures "d50" distance of L12.start P1
  measures "d51" distance of L18.start P2
  measures "d52" distance of L24.start P3
  measures "d53" distance of L30.start P4
  measures "d54" distance of L36.start P5
  measures "d55" distance of L42.start P6
  measures "d56" distance of L48.start P7
extrude "Extrude2" cut sketch "Sketch5" against normal blind 2.2 contours L0 L2 L42 L44 L45 L46 L47 | L0 L42 L43 L44 | L2 L42 L47 | L1 L51 L52 L53 | L1 L2 L48 L49 L50 L51 L53 | L2 L48 L53 | L0 L36 L38 L39 L40 L41 | L0 L36 L37 L38 | L1 L33 L34 L35 | L1 L30 L31 L32 L33 L35 | L0 L18 L19 L20 L21 L23 | L0 L21 L22 L23 | L1 L24 L25 L26 | L1 L24 L26 L27 L28 L29 | L0 L12 L14 L15 L16 L17 | L0 L12 L13 L14 | L1 L9 L10 L11 | L1 L6 L7 L8 L9 L11 | A0 | A2 | A5 | A10 | A11 | A12 | A17 | A23 bodies 2
extrude "Extrude3" add 1 faces at (19.25, 10.55, 40.25) along direction (0, 0, 1) blind 0.1 on bodies 2 bodies 2
extrude "Extrude4" add 1 faces at (19.25, 10.55, 0) along direction (0, 0, -1) blind 0.1 on bodies 2 bodies 2
delete_face "DeleteFace1" 1 faces at (4.6214, 2.6716, 19.2813) on bodies 2
delete_face "DeleteFace2" 1 faces at (27.1286, 2.6716, 19.2813) on bodies 2
hidden bodies 1
equation "frame_width_Ref = 31.75 mm"
equation "frame_dist_base_screw_Ref = 5.0313 mm"
equation "frame_dist_scew_screw_Ref = 10.0625 mm"
equation "frame_heatinst_diameter_Ref = 4 mm"
equation "frame_align_top_offset_maj_Ref = 0.9 mm"
equation "frame_align_top_off_min_Ref = 0.65 mm"
equation "frame_4_height_Ref = 261.625 mm"
equation "frame_side_offset_Ref = 4.25 mm"
equation "frame_thick_min_Ref = 2 mm"
equation "frame_dia_screw_struct_Ref = 6.2 mm"
equation "frame_align_height_Ref = 3.05 mm"
equation "d17 = frame_dist_scew_screw_Ref * 4"
